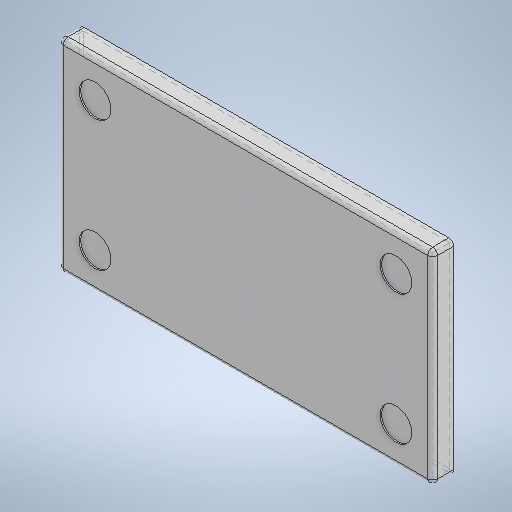
# Autodesk Inventor part: Datapad_Case_v2
Saved by Autodesk Inventor 2025 (Build 290162000, 162)
## iProperties
Created: 2026-06-22
Part Number: Datapad_Case_v2
Material: Generisch
Document SubType Name: Modeling
Designer: plauffs
Density: 1 g/cm^3
Appearance: Vorgabe
Author: plauffs
Autodesk Inventor part; units mm, degrees
ref_plane "YZ Plane" through (0, 0, 0) normal (1, 0, 0) x (0, 1, 0)
ref_plane "XZ Plane" through (0, 0, 0) normal (0, 1, 0) x (-1, 0, 0)
ref_plane "XY Plane" through (0, 0, 0) normal (0, 0, 1) x (1, 0, 0)
sketch "Skizze1" plane through (0, 0, 0) normal (0, 1, 0) x (-1, 0, 0)
  line L0 (0, 0) -> (153.2, 0)
  line L1 (153.2, 0) -> (153.2, -83.2)
  line L2 (153.2, -83.2) -> (0, -83.2)
  line L3 (0, -83.2) -> (0, 0)
  dimension "d0" = 153.2
  dimension "d1" = 83.2
  constraints: 8 end point, 2 parallel, 1 horizontal, 1 perpendicular
  measures "d0" distance of L1.end L2.end
  measures "d1" distance of L0.end L1.end
extrude "Extrusion1" add sketch "Skizze1" along normal blind 8.6
sketch "Skizze2" plane through (0, 8.6, 0) normal (0, 1, 0) x (1, 0, 0)
  line L0 (-1.5, 1.5) -> (-151.7, 1.5)
  line L1 (-151.7, 1.5) -> (-151.7, 81.7)
  line L2 (-151.7, 81.7) -> (-1.5, 81.7)
  line L3 (-1.5, 81.7) -> (-1.5, 1.5)
  line L4 (-153.2, 0) -> (0, 0) projected
  line L5 (0, 83.2) -> (-153.2, 83.2) projected
  line L6 (0, 0) -> (0, 83.2) projected
  line L7 (-153.2, 83.2) -> (-153.2, 0) projected
  dimension "d4" = 1.5
  dimension "d5" = 1.5
  dimension "d6" = 1.5
  dimension "d7" = 1.5
  constraints: 8 end point, 2 parallel, 1 horizontal, 1 perpendicular
  measures "d4" distance between parallel lines of L4 L0
  measures "d5" distance between parallel lines of L5 L2
  measures "d6" distance between parallel lines of L6 L3
  measures "d7" distance between parallel lines of L7 L1
extrude "Extrusion2" cut sketch "Skizze2" against normal blind 7.1 contours L0 L1 L2 L3
sketch "Skizze4" plane through (0, 1.5, 0) normal (0, 1, 0) x (1, 0, 0)
  circle A0 centre (-80.05, 22.6) radius 2.75
  circle A1 centre (-80.05, 60.6) radius 2.75
  circle A2 centre (-23.05, 22.6) radius 2.75
  circle A3 centre (-23.05, 60.6) radius 2.75
  circle A4 centre (-80.05, 22.6) radius 1.2
  circle A5 centre (-80.05, 60.6) radius 1.2
  circle A6 centre (-23.05, 22.6) radius 1.2
  circle A7 centre (-23.05, 60.6) radius 1.2
  line L0 (-1.5, 81.7) -> (-1.5, 1.5) projected
  line L1 (-1.5, 1.5) -> (-151.7, 1.5) projected
  line L2 (-151.7, 81.7) -> (-1.5, 81.7) projected
  point P0 (0, 0)
  dimension "d13" = 5.5
  dimension "d14" = 5.5
  dimension "d15" = 5.5
  dimension "d16" = 5.5
  dimension "d17" = 38
  dimension "d18" = 38
  dimension "d19" = 57
  dimension "d40" = 2.4
  dimension "d41" = 2.4
  dimension "d42" = 2.4
  dimension "d43" = 2.4
  dimension "d44" = 21.55
  dimension "d45" = 21.1
  dimension "d47" = 21.1
  dimension "d51" = 21.55
  dimension "d53" = 57
  dimension "d54" = 21.1
  dimension "d55" = 21.1
  constraints: 8 centre point, 4 coincident
  measures "d13" diameter of A0
  measures "d14" diameter of A1
  measures "d15" diameter of A2
  measures "d16" diameter of A3
  measures "d17" distance of A1.centre A0.centre
  measures "d18" distance of A3.centre A2.centre
  measures "d19" distance of A2.centre A0.centre
  measures "d40" diameter of A4
  measures "d41" diameter of A5
  measures "d42" diameter of A6
  measures "d43" diameter of A7
  measures "d44" distance from line of L0 A2.centre
  measures "d45" distance from line of L1 A0.centre
  measures "d47" distance from line of L1 A2.centre
  measures "d51" distance from line of L0 A3.centre
  measures "d53" distance of A3.centre A1.centre
  measures "d54" distance from line of L2 A3.centre
  measures "d55" distance from line of L2 A5.centre
extrude "Extrusion4" add sketch "Skizze4" along normal blind 5.5
fillet "Rundung1" radius 2 4 edges at (0, 4.3, 0) (0, 4.3, -83.2) (-153.2, 4.3, 0) (-153.2, 4.3, -83.2)
fillet "Rundung2" radius 2 8 edges at (-0.5858, 0, -0.5858) (0, 0, -41.6) (-0.5858, 0, -82.6142) (-76.6, 0, -83.2) (-152.6142, 0, -82.6142) (-153.2, 0, -41.6) (-152.6142, 0, -0.5858) (-76.6, 0, 0)
sketch "Skizze6" plane through (0, 0, 0) normal (0, -1, 0) x (1, 0, 0)
  circle A0 centre (-138.2, -68.2) radius 6.5
  circle A1 centre (-138.2, -15) radius 6.5
  circle A2 centre (-15, -68.2) radius 6.5
  circle A3 centre (-15, -15) radius 6.5
  line L0 (-2, 0) -> (-151.2, 0) projected
  line L1 (-151.2, -83.2) -> (-2, -83.2) projected
  line L2 (-153.2, -2) -> (-153.2, -81.2) projected
  line L3 (0, -81.2) -> (0, -2) projected
  point P0 (0, 0)
  dimension "d26" = 13
  dimension "d27" = 13
  dimension "d28" = 13
  dimension "d29" = 13
  dimension "d63" = 15
  dimension "d64" = 15
  dimension "d65" = 15
  dimension "d66" = 15
  dimension "d67" = 15
  dimension "d68" = 15
  dimension "d69" = 15
  dimension "d70" = 15
  constraints: 4 centre point
  measures "d26" diameter of A0
  measures "d27" diameter of A1
  measures "d28" diameter of A2
  measures "d29" diameter of A3
  measures "d63" distance from line of L0 A1.centre
  measures "d64" distance from line of L1 A0.centre
  measures "d65" distance from line of L0 A3.centre
  measures "d66" distance from line of L1 A2.centre
  measures "d67" distance from line of L2 A0.centre
  measures "d68" distance from line of L2 A1.centre
  measures "d69" distance from line of L3 A2.centre
  measures "d70" distance from line of L3 A3.centre
extrude "Extrusion6" cut sketch "Skizze6" against normal blind 0.6
